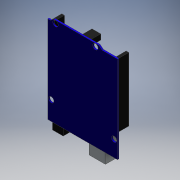
# Autodesk Inventor part: arduino uno
Saved by Autodesk Inventor 2016 (Build 200138000, 138)
## iProperties
Created: 2017-12-27
Part Number: arduino uno
Material: Genérico
Document SubType Name: Sheet Metal
Designer: David
Density: 1 g/cm^3
Sheet Metal Rule: Por defecto_mm
Appearance: Valor por defecto
Author: David
Autodesk Inventor part; units mm, degrees
ref_plane "YZ Plane" through (0, 0, 0) normal (1, 0, 0) x (0, 1, 0)
ref_plane "XZ Plane" through (0, 0, 0) normal (0, 1, 0) x (-1, 0, 0)
ref_plane "XY Plane" through (0, 0, 0) normal (0, 0, 1) x (1, 0, 0)
sketch "Boceto1" plane through (0, 0, 0) normal (0, 1, 0) x (-1, 0, 0)
  line L0 (-52, -2) -> (-52, -55)
  line L1 (-52, -67) -> (0, -67)
  line L2 (0, -67) -> (0, -2)
  line L3 (-52, -2) -> (-40.5, -2)
  line L4 (-40.5, -2) -> (-38, 0)
  line L5 (-38, 0) -> (-4.5, 0)
  line L6 (0, -2) -> (-2, -2)
  line L7 (-4.5, 0) -> (-2, -2)
  line L8 (-52, -67) -> (-52, -55)
  circle A0 centre (-49.4429, -55) radius 2
  circle A1 centre (-2.5817, -53) radius 2
  circle A2 centre (-35.5, -2.2598) radius 2
  line L9 (-4.5, 0) -> (-7, 0)
  circle A3 centre (-5.75, -2.2598) radius 2
  point P0 (0, 0)
  constraints: 20 end point, 4 centre point, 4 point on line, 1 horizontal, 1 parallel
extrude "Extrusión1" add sketch "Boceto1" along normal blind 1
sketch "Boceto2" plane through (0, 1, 0) normal (0, 1, 0) x (1, 0, 0)
  line L0 (49, 3) -> (51, 3)
  line L1 (51, 3) -> (51, 50.5)
  line L2 (40.5, 2) -> (52, 2) projected
  line L3 (52, 2) -> (52, 67) projected
  line L4 (49, 3) -> (49, 50.5)
  line L5 (49, 50.5) -> (51, 50.5)
  line L6 (1.1059, 3) -> (3, 3)
  line L7 (0, 2) -> (2, 2) projected
  line L8 (0, 67) -> (0, 2) projected
  line L9 (1.1059, 3) -> (1, 3)
  line L10 (1, 3) -> (1, 41)
  line L11 (1, 41) -> (3.1059, 41)
  line L12 (3, 41) -> (3, 3)
  point P0 (0, 0)
  constraints: 18 end point, 3 horizontal, 1 point on line
extrude "Extrusión2" add sketch "Boceto2" along normal blind 8.45
sketch "Boceto3" plane through (0, 1, 0) normal (0, 1, 0) x (1, 0, 0)
  line L0 (30.5, 1) -> (30.5, 5)
  line L1 (24, 1) -> (24, 5)
  line L2 (24, 5) -> (30.5, 5)
  line L3 (30.5, 1) -> (24, 1)
  point P0 (0, 0)
  point P1 (38, 0)
  constraints: 8 end point, 1 horizontal, 1 perpendicular, 1 vertical
extrude "Extrusión3" add sketch "Boceto3" along normal blind 8
sketch "Boceto4" plane through (0, 1, 0) normal (0, 1, 0) x (1, 0, 0)
  line L0 (42, 67) -> (42, 59.5)
  line L1 (42, 59.5) -> (30, 59.5)
  line L2 (30, 59.5) -> (30, 75.5)
  line L3 (30, 75.5) -> (42, 75.5)
  line L4 (42, 75.5) -> (42, 67)
  point P0 (0, 0)
  point P1 (52, 67)
  constraints: 10 end point, 2 horizontal, 2 vertical, 1 collinear
extrude "Extrusión4" add sketch "Boceto4" along normal blind 10
sketch "Boceto5" plane through (0, 1, 0) normal (0, 1, 0) x (1, 0, 0)
  line L0 (2.5, 67) -> (2.5, 59)
  line L1 (2.5, 59) -> (10.5, 59)
  line L2 (10.5, 59) -> (10.5, 73)
  line L3 (10.5, 73) -> (2.5, 73)
  line L4 (2.5, 73) -> (2.5, 67)
  point P0 (0, 0)
  point P1 (0, 67)
  constraints: 10 end point, 2 vertical, 1 horizontal
extrude "Extrusión5" add sketch "Boceto5" along normal blind 10
sketch "Boceto6" plane through (2.5, 1, -59) normal (0, 0, 1) x (1, 0, 0)
  line L0 (0, 10) -> (8, 10) projected
  arc A0 (7.8719, 6) -> (0.1281, 6) centre (4, 6) ccw
  line L1 (8, 0) -> (8, 10) projected
  line L2 (0, 6) -> (0.1281, 6)
  line L3 (7.8719, 6) -> (8, 6)
  line L4 (8, 6) -> (8, 10)
  line L5 (0, 10) -> (8, 10)
  line L6 (0, 0) -> (0, 10) projected
  line L7 (0, 10) -> (0, 6)
  point P0 (-2.5, -1)
  constraints: 10 end point, 2 collinear, 2 horizontal, 2 point on circle, 1 centre point, 1 perpendicular, 1 point on line
extrude "Extrusión6" cut sketch "Boceto6" against normal blind 12
equation "\"Radio_pliegue\" = Grosor"
equation "\"Anchura_desahogo_plegado\" = Grosor"
equation "\"Profundidad_desahogo_plegado\" = 0.5 * Grosor"
equation "\"Tamaño_destalonado\" = 4 * Grosor"
equation "\"Remanente_mínimo\" = 2 * Grosor"
equation "\"Radiodetransición\" = Radio_pliegue"
equation "\"Tamaño_de_radio_de_Jacobi\" = Radio_pliegue"
equation "\"TamañoSeparación\" = Grosor"
equation "\"Grosor\" = 0.5"
